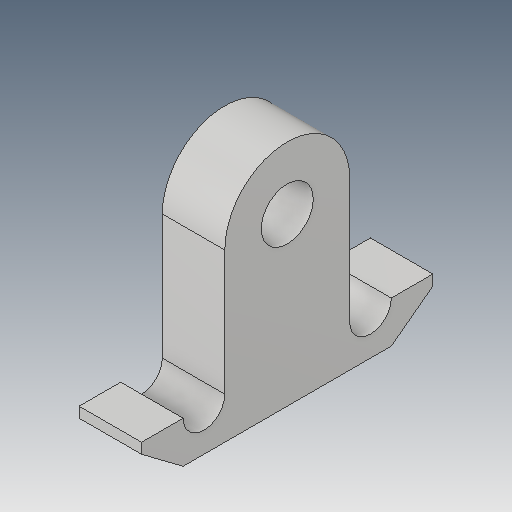
# Autodesk Inventor part: tip3
Saved by Autodesk Inventor 2019.4 (Build 234330000, 330)
## iProperties
Created: 2019-06-11
Part Number: tip3
Material: アルミニウム 2014-T4
Document SubType Name: Modeling
Designer: AzLIer
Density: 2.8 g/cm^3
Appearance: サテン
Mass: 0.563529 g
Surface Area: 3.0086 cm^2
Volume: 0.201261 cm^3
Author: AzLIer
Autodesk Inventor part; units mm, degrees
ref_plane "YZ Plane" through (0, 0, 0) normal (1, 0, 0) x (0, 1, 0)
ref_plane "XZ Plane" through (0, 0, 0) normal (0, 1, 0) x (-1, 0, 0)
ref_plane "XY Plane" through (0, 0, 0) normal (0, 0, 1) x (1, 0, 0)
sketch "スケッチ1" plane through (0, 0, 0) normal (1, 0, 0) x (0, 1, 0)
  line L0 (9, 0) -> (-9, 0) construction
  line L1 (9, 3) -> (-9, 3)
  line L2 (-9, -3) -> (9, -3)
  arc A0 (9, -3) -> (9, 3) centre (9, 0) ccw
  arc A1 (-9, 3) -> (-9, -3) centre (-9, 0) ccw
  line L3 (3, 7) -> (-3, 7)
  line L4 (-3, -7) -> (3, -7)
  line L5 (3, 7) -> (-3, -7) construction
  line L6 (-3, 7) -> (3, -7) construction
  line L7 (-3, 7) -> (-3, 5)
  line L8 (3, 5) -> (3, 7)
  line L9 (3, -7) -> (3, -5)
  line L10 (3, -3) -> (3, 3)
  line L11 (-3, 3) -> (-3, -3)
  line L12 (-3, -5) -> (-3, -7)
  circle A2 centre (-9, 0) radius 1.25
  circle A3 centre (9, 0) radius 1.25
  line L13 (3, -5) -> (3, -3)
  line L14 (3, 3) -> (3, 5)
  line L15 (-3, 5) -> (-3, 3)
  line L16 (-3, -3) -> (-3, -5)
  point P0 (0, 0)
  dimension "d0" = 6
  dimension "d1" = 6
  dimension "d3" = 14
  dimension "d4" = 18
  dimension "d7" = 0
  dimension "d8" = 6
  dimension "d9" = 4
  dimension "d11" = 2.5
  dimension "d12" = 2.5
  constraints: 36 end point, 12 parallel, 4 centre point, 4 collinear, 4 point on circle, 4 tangent, 3 midpoint, 3 perpendicular, 2 coincident, 2 horizontal, 2 point on line
  measures "d0" diameter of A1
  measures "d1" distance of L4.start L4.end
  measures "d3" distance between parallel lines of L4 L3
  measures "d4" distance of L0.start L0.end
  measures "d7" distance between parallel lines of L8 L10
  measures "d8" distance between parallel lines of L8 L11
  measures "d9" distance from line of L10.start L4
  measures "d11" diameter of A2
  measures "d12" diameter of A3
extrude "押し出し1" add sketch "スケッチ1" along normal blind 3 contours A0 L2 L10 L1 | L10 L2 L11 L1 | L1 L15 L7 L3 L8 L14 | L11 L2 A1 L1 | L13 L9 L4 L12 L16 L2 | A2 | A3
sketch "スケッチ2" plane through (0, 0, 0) normal (-1, 0, 0) x (0, 0, 1)
  circle A0 centre (0, 9) radius 1.25 projected
  circle A1 centre (0, -9) radius 1.25 projected
  line L0 (-3, 3) -> (-7, 3) projected
  line L1 (-7, 3) -> (-7, -3) projected
  line L2 (-7, -3) -> (-3, -3) projected
  line L3 (-3, -3) -> (-3, -9) projected
  arc A2 (-3, -9) -> (3, -9) centre (0, -9) ccw projected
  line L4 (3, -9) -> (3, -3) projected
  line L5 (3, -3) -> (7, -3) projected
  line L6 (7, -3) -> (7, 3) projected
  line L7 (7, 3) -> (3, 3) projected
  line L8 (3, 3) -> (3, 9) projected
  arc A3 (3, 9) -> (-3, 9) centre (0, 9) ccw projected
  line L9 (-3, 9) -> (-3, 3) projected
  line L10 (-7, 2.5) -> (-5, 1)
  line L11 (-5, 1) -> (5, 1)
  line L12 (5, 1) -> (7, 2.5)
  line L13 (3, 3) -> (3, 9) projected
  line L14 (-3, 9) -> (-3, 3) projected
  arc A4 (-5, 3) -> (-3, 3) centre (-4, 3) ccw
  arc A5 (3, 3) -> (5, 3) centre (4, 3) ccw
  point P0 (0, 0)
  point P1 (0, 1)
  dimension "d17" = 10
  dimension "d18" = 2
  dimension "d19" = 0.5
  dimension "d26" = 2
  constraints: 9 end point, 4 point on circle, 4 point on line, 3 midpoint, 2 centre point, 1 equal length, 1 equal radius, 1 horizontal, 1 vertical alignment
  measures "d17" distance of L10.end L11.end
  measures "d18" distance between parallel lines of L0 L11
  measures "d19" distance from line of L0 L10.start
  measures "d26" diameter of A4
extrude "押し出し4" cut sketch "スケッチ2" against normal through all contours L9 A3 L8 A5 L7 L6 L12 L11 L10 L1 L0 A4 keep common part
